Autodesk Fusion 360 part; units mm, degrees
note: some values were not read from the file. Set by a fixed rule: which sketch regions a step uses.
(part 2 of 2)
  spline S201 degree 3 poles (6.8488, 8.7661) (6.8423, 8.7918) (6.8421, 8.8259) (6.8482, 8.842) knots 0 0 0 0 1 1 1 1
  spline S202 degree 3 poles (8.7414, 7.2125) (8.7777, 7.2173) (8.7826, 7.2354) (8.7879, 7.3852) knots 0 0 0 0 1 1 1 1
  spline S203 degree 3 poles (9.5315, 7.0264) (9.6667, 6.9334) (9.8914, 6.6784) (9.9898, 6.5065) knots 0 0 0 0 1 1 1 1
  spline S204 degree 3 poles (9.748, 4.1018) (9.7258, 4.0149) (9.6698, 3.8347) (9.6236, 3.7012) knots 0 0 0 0 1 1 1 1
  spline S205 degree 3 poles (9.605, 10.5653) (9.605, 10.4649) (9.5312, 10.3126) (9.4656, 10.2775) knots 0 0 0 0 1 1 1 1
  spline S206 degree 3 poles (1.6447, 7.4321) (1.665, 7.8082) (1.7553, 8.1252) (1.9194, 8.3954) knots 0 0 0 0 1 1 1 1
  spline S207 degree 3 poles (9.5653, 3.7025) (9.6095, 3.8254) (9.6666, 4.0083) (9.6922, 4.1089) knots 0 0 0 0 1 1 1 1
  spline S208 degree 3 poles (9.4532, 3.3234) (9.4707, 3.409) (9.5212, 3.5795) (9.5653, 3.7025) knots 0 0 0 0 1 1 1 1
  spline S209 degree 3 poles (7.2255, 1.1728) (7.0951, 1.1191) (7.0078, 1.066) (6.9157, 0.9846) knots 0 0 0 0 1 1 1 1
  spline S210 degree 3 poles (10.2177, 5.0639) (10.1598, 4.8501) (10.0228, 4.569) (9.8929, 4.3977) knots 0 0 0 0 1 1 1 1
  spline S211 degree 3 poles (8.0403, 1.7091) (8.1353, 1.7773) (8.2598, 1.8521) (8.3169, 1.8754) knots 0 0 0 0 1 1 1 1
  spline S212 degree 3 poles (8.3787, 8.4165) (8.1204, 8.6765) (7.8311, 8.8118) (7.451, 8.8504) knots 0 0 0 0 1 1 1 1
  spline S213 degree 3 poles (8.0122, 1.6173) (7.7401, 1.4262) (7.4702, 1.2738) (7.2255, 1.1728) knots 0 0 0 0 1 1 1 1
  spline S214 degree 3 poles (1.4592, 7.0165) (1.6041, 7.1229) (1.6313, 7.1838) (1.6447, 7.4321) knots 0 0 0 0 1 1 1 1
  spline S215 degree 3 poles (6.8967, 8.8154) (6.8438, 8.7625) (7.1598, 8.3823) (7.5375, 8.0447) knots 0 0 0 0 1 1 1 1
  spline S216 degree 3 poles (9.404, 10.1458) (9.3772, 10.0264) (9.2567, 9.8669) (9.1498, 9.8097) knots 0 0 0 0 1 1 1 1
  spline S217 degree 3 poles (7.451, 8.8504) (7.2485, 8.871) (6.9323, 8.851) (6.8967, 8.8154) knots 0 0 0 0 1 1 1 1
  spline S218 degree 3 poles (2.0429, 7.257) (2.0099, 7.3294) (2.0562, 7.7293) (2.1195, 7.9187) knots 0 0 0 0 1 1 1 1
  spline S219 degree 3 poles (9.3549, 7.4617) (9.369, 7.1961) (9.4015, 7.1158) (9.5315, 7.0264) knots 0 0 0 0 1 1 1 1
  spline S220 degree 3 poles (8.7879, 7.3852) (8.7955, 7.6006) (8.7375, 7.8504) (8.6269, 8.0792) knots 0 0 0 0 1 1 1 1
  line L42 (8.5585, 7.2249) -> (8.5585, 7.2249)
  spline S221 degree 3 poles (9.7891, 11.6914) (9.7747, 11.6536) (9.7797, 11.6222) (9.8094, 11.5639) knots 0 0 0 0 1 1 1 1
  spline S222 degree 3 poles (9.1498, 9.8097) (9.1159, 9.7916) (9.0876, 9.7515) (9.0721, 9.6998) knots 0 0 0 0 1 1 1 1
  spline S223 degree 3 poles (2.481, 8.5) (2.6158, 8.635) (2.6801, 8.6816) (2.8384, 8.759) knots 0 0 0 0 1 1 1 1
  spline S224 degree 3 poles (10.2182, 5.9527) (10.2797, 5.7253) (10.2795, 5.292) (10.2177, 5.0639) knots 0 0 0 0 1 1 1 1
  line L43 (2.0249, 10.215) -> (2.1125, 10.2252)
  line L44 (5.7675, 7.7349) -> (5.7675, 7.7349)
  spline S225 degree 3 poles (1.477, 11.3964) (1.477, 11.406) (1.5272, 11.4139) (1.5887, 11.4139) knots 0 0 0 0 1 1 1 1
  spline S226 degree 3 poles (5.1964, 5.9716) (5.0404, 5.426) (4.5977, 4.9756) (4.075, 4.8308) knots 0 0 0 0 1 1 1 1
  spline S227 degree 3 poles (4.3387, 8.5706) (4.0922, 8.182) (4.6976, 7.738) (5.5003, 7.7186) knots 0 0 0 0 1 1 1 1
  spline S228 degree 3 poles (2.6301, 9.5918) (2.4593, 9.6417) (2.2491, 9.7435) (2.2491, 9.7763) knots 0 0 0 0 1 1 1 1
  spline S229 degree 3 poles (5.7675, 7.7349) (6.1571, 7.7759) (6.45, 7.8899) (6.6031, 8.0602) knots 0 0 0 0 1 1 1 1
  spline S230 degree 3 poles (2.003, 10.3004) (1.7807, 10.4532) (1.6559, 10.6247) (1.7891, 10.5945) knots 0 0 0 0 1 1 1 1
  spline S231 degree 3 poles (5.0939, 9.0802) (4.7717, 8.9797) (4.4682, 8.7749) (4.3387, 8.5706) knots 0 0 0 0 1 1 1 1
  spline S232 degree 3 poles (1.7972, 10.7093) (1.6781, 10.811) (1.5786, 10.9388) (1.5786, 10.9899) knots 0 0 0 0 1 1 1 1
  spline S233 degree 3 poles (5.0735, 5.7716) (5.1562, 5.9541) (5.1945, 6.1138) (5.208, 6.3339) knots 0 0 0 0 1 1 1 1
  spline S234 degree 3 poles (4.0117, 4.8607) (4.4627, 4.9671) (4.8653, 5.3124) (5.0735, 5.7716) knots 0 0 0 0 1 1 1 1
  spline S235 degree 3 poles (5.208, 6.3339) (5.2458, 6.9461) (4.8768, 7.4468) (4.3151, 7.5455) knots 0 0 0 0 1 1 1 1
  spline S236 degree 3 poles (4.3151, 7.5455) (4.1262, 7.5787) (3.9908, 7.5694) (3.7838, 7.5092) knots 0 0 0 0 1 1 1 1
  spline S237 degree 3 poles (8.2433, 6.7505) (8.3487, 6.5329) (8.3856, 6.3861) (8.3997, 6.1287) knots 0 0 0 0 1 1 1 1
  spline S238 degree 3 poles (7.5116, 7.5114) (7.8229, 7.3495) (8.0852, 7.0767) (8.2433, 6.7505) knots 0 0 0 0 1 1 1 1
  spline S239 degree 3 poles (2.2593, 9.929) (2.0696, 10.0329) (1.9188, 10.1485) (1.9297, 10.1816) knots 0 0 0 0 1 1 1 1
  spline S240 degree 3 poles (5.8117, 6.8927) (6.0456, 7.6034) (6.8041, 7.8795) (7.5116, 7.5114) knots 0 0 0 0 1 1 1 1
  spline S241 degree 3 poles (5.5003, 7.7186) (5.5506, 7.7174) (5.6708, 7.7247) (5.7675, 7.7349) knots 0 0 0 0 1 1 1 1
  spline S242 degree 3 poles (3.7122, 4.831) (3.8072, 4.8309) (3.942, 4.8443) (4.0117, 4.8607) knots 0 0 0 0 1 1 1 1
  spline S243 degree 3 poles (1.7003, 11.4393) (1.7, 11.4746) (1.6076, 11.6698) (1.5583, 11.7389) knots 0 0 0 0 1 1 1 1
  spline S244 degree 3 poles (8.3997, 6.1287) (8.4213, 5.7357) (8.311, 5.4218) (8.0651, 5.1759) knots 0 0 0 0 1 1 1 1
  spline S245 degree 3 poles (4.279, 8.5648) (4.3224, 8.6498) (4.4952, 8.8262) (4.6141, 8.9068) knots 0 0 0 0 1 1 1 1
  spline S246 degree 3 poles (8.0651, 5.1759) (7.7847, 4.8955) (7.4026, 4.7916) (6.9851, 4.8821) knots 0 0 0 0 1 1 1 1
  spline S247 degree 3 poles (7.8704, 7.193) (7.1638, 7.8887) (6.1547, 7.7346) (5.8598, 6.8859) knots 0 0 0 0 1 1 1 1
  spline S248 degree 3 poles (8.3349, 5.7751) (8.4358, 6.2558) (8.2518, 6.8174) (7.8704, 7.193) knots 0 0 0 0 1 1 1 1
  spline S249 degree 3 poles (6.6831, 8.5182) (6.5678, 8.7465) (6.2355, 8.9773) (5.872, 9.0815) knots 0 0 0 0 1 1 1 1
  spline S250 degree 3 poles (2.0867, 7.5233) (2.0579, 7.2435) (2.0842, 7.2071) (2.2619, 7.281) knots 0 0 0 0 1 1 1 1
  spline S251 degree 3 poles (6.7094, 8.5665) (6.7799, 8.4383) (6.7915, 8.2563) (6.7359, 8.1525) knots 0 0 0 0 1 1 1 1
  spline S252 degree 3 poles (2.7063, 9.5038) (2.7343, 9.5144) (2.7571, 9.5302) (2.7571, 9.5389) knots 0 0 0 0 1 1 1 1
  spline S253 degree 3 poles (6.7359, 8.1525) (6.5514, 7.8081) (5.9013, 7.6142) (5.2158, 7.6991) knots 0 0 0 0 1 1 1 1
  spline S254 degree 3 poles (2.7571, 9.5389) (2.7571, 9.5475) (2.6999, 9.5713) (2.6301, 9.5918) knots 0 0 0 0 1 1 1 1
  spline S255 degree 3 poles (1.9297, 10.1816) (1.9339, 10.1944) (1.9767, 10.2094) (2.0249, 10.215) knots 0 0 0 0 1 1 1 1
  spline S256 degree 3 poles (5.1947, 9.1494) (5.4148, 9.1938) (5.7145, 9.1806) (5.9169, 9.1174) knots 0 0 0 0 1 1 1 1
  spline S257 degree 3 poles (2.2491, 9.7763) (2.2491, 9.7911) (2.2874, 9.8111) (2.3355, 9.8214) knots 0 0 0 0 1 1 1 1
  spline S258 degree 3 poles (5.9169, 9.1174) (6.2615, 9.0098) (6.592, 8.7801) (6.7094, 8.5665) knots 0 0 0 0 1 1 1 1
  spline S259 degree 3 poles (1.5887, 11.4139) (1.6647, 11.4139) (1.7004, 11.422) (1.7003, 11.4393) knots 0 0 0 0 1 1 1 1
  spline S260 degree 3 poles (3.7934, 7.5652) (3.9997, 7.6214) (4.3135, 7.6144) (4.4966, 7.5495) knots 0 0 0 0 1 1 1 1
  spline S261 degree 3 poles (5.2283, 6.6997) (5.2698, 6.5029) (5.2557, 6.1786) (5.1964, 5.9716) knots 0 0 0 0 1 1 1 1
  spline S262 degree 3 poles (1.698, 11.1132) (1.5887, 11.2162) (1.477, 11.3594) (1.477, 11.3964) knots 0 0 0 0 1 1 1 1
  spline S263 degree 3 poles (4.4966, 7.5495) (4.8766, 7.4147) (5.1424, 7.106) (5.2283, 6.6997) knots 0 0 0 0 1 1 1 1
  spline S264 degree 3 poles (4.075, 4.8308) (3.9008, 4.7825) (3.5773, 4.7772) (3.4214, 4.8201) knots 0 0 0 0 1 1 1 1
  spline S265 degree 3 poles (3.9654, 8.7696) (4.0196, 8.8762) (3.9969, 8.8841) (3.635, 8.8841) knots 0 0 0 0 1 1 1 1
  spline S266 degree 3 poles (6.6031, 8.0602) (6.7405, 8.213) (6.7654, 8.3552) (6.6831, 8.5182) knots 0 0 0 0 1 1 1 1
  spline S267 degree 3 poles (3.7838, 7.5092) (3.1288, 7.3184) (2.6508, 6.6827) (2.6479, 5.9986) knots 0 0 0 0 1 1 1 1
  spline S268 degree 3 poles (2.7689, 5.4275) (2.9421, 5.0611) (3.3051, 4.8316) (3.7122, 4.831) knots 0 0 0 0 1 1 1 1
  spline S269 degree 3 poles (1.5786, 10.9899) (1.5786, 11.0151) (1.6007, 11.0195) (1.6954, 11.0133) knots 0 0 0 0 1 1 1 1
  spline S270 degree 3 poles (2.6479, 5.9986) (2.6469, 5.76) (2.6754, 5.6251) (2.7689, 5.4275) knots 0 0 0 0 1 1 1 1
  spline S271 degree 3 poles (5.802, 6.0703) (5.7337, 6.3243) (5.7377, 6.668) (5.8117, 6.8927) knots 0 0 0 0 1 1 1 1
  spline S272 degree 3 poles (6.9851, 4.8821) (6.4518, 4.9978) (5.9569, 5.4948) (5.802, 6.0703) knots 0 0 0 0 1 1 1 1
  spline S273 degree 3 poles (3.1867, 9.2589) (3.2684, 9.3193) (3.2462, 9.3318) (3.0249, 9.3504) knots 0 0 0 0 1 1 1 1
  spline S274 degree 3 poles (4.5847, 7.9094) (4.4511, 7.9906) (4.3109, 8.1351) (4.2694, 8.2344) knots 0 0 0 0 1 1 1 1
  spline S275 degree 3 poles (3.635, 8.8841) (3.3624, 8.8841) (3.2924, 8.8773) (3.1545, 8.8373) knots 0 0 0 0 1 1 1 1
  spline S276 degree 3 poles (3.0249, 9.3504) (2.7221, 9.3759) (2.5667, 9.4507) (2.7063, 9.5038) knots 0 0 0 0 1 1 1 1
  spline S277 degree 3 poles (4.6141, 8.9068) (4.7582, 9.0046) (5.0205, 9.1142) (5.1947, 9.1494) knots 0 0 0 0 1 1 1 1
  spline S278 degree 3 poles (4.2694, 8.2344) (4.2291, 8.3308) (4.2333, 8.4754) (4.279, 8.5648) knots 0 0 0 0 1 1 1 1
  spline S279 degree 3 poles (5.2158, 7.6991) (5.0217, 7.7232) (4.7329, 7.8194) (4.5847, 7.9094) knots 0 0 0 0 1 1 1 1
  spline S280 degree 3 poles (3.1584, 9.1724) (3.1077, 9.1856) (3.1141, 9.2052) (3.1867, 9.2589) knots 0 0 0 0 1 1 1 1
  spline S281 degree 3 poles (1.7891, 10.5945) (1.813, 10.5891) (1.8498, 10.5912) (1.8708, 10.5992) knots 0 0 0 0 1 1 1 1
  line L45 (2.3355, 9.8214) -> (2.4218, 9.84)
  line L46 (2.4218, 9.84) -> (2.2593, 9.929)
  spline S282 degree 3 poles (5.872, 9.0815) (5.6441, 9.1468) (5.3056, 9.1463) (5.0939, 9.0802) knots 0 0 0 0 1 1 1 1
  spline S283 degree 3 poles (1.8708, 10.5992) (1.9038, 10.6117) (1.8936, 10.6269) (1.7972, 10.7093) knots 0 0 0 0 1 1 1 1
  line L47 (2.1125, 10.2252) -> (2.003, 10.3004)
  spline S284 degree 3 poles (1.2763, 4.8425) (1.0557, 5.2885) (1.0727, 5.8763) (1.318, 6.288) knots 0 0 0 0 1 1 1 1
  spline S285 degree 3 poles (4.2059, 3.3632) (4.1426, 3.5277) (4.1196, 3.8574) (4.1584, 4.0441) knots 0 0 0 0 1 1 1 1
  spline S286 degree 3 poles (4.1795, 1.601) (4.1795, 1.5168) (4.292, 1.3626) (4.4437, 1.2387) knots 0 0 0 0 1 1 1 1
  spline S287 degree 3 poles (8.7941, 4.5029) (8.5375, 4.6444) (8.1575, 4.4807) (7.7149, 4.0381) knots 0 0 0 0 1 1 1 1
  spline S288 degree 3 poles (1.8517, 3.8425) (1.9024, 4.3071) (2.1479, 4.4859) (2.5803, 4.3732) knots 0 0 0 0 1 1 1 1
  spline S289 degree 3 poles (5.1369, 0.8861) (5.3563, 0.8305) (5.6964, 0.8433) (5.9169, 0.9154) knots 0 0 0 0 1 1 1 1
  spline S290 degree 3 poles (3.8769, 2.6151) (3.876, 3.0027) (3.6864, 3.4542) (3.3879, 3.7794) knots 0 0 0 0 1 1 1 1
  spline S291 degree 3 poles (7.7149, 4.0381) (7.3234, 3.6464) (7.1023, 3.2168) (7.0405, 2.7271) knots 0 0 0 0 1 1 1 1
  spline S292 degree 3 poles (5.8166, 2.5154) (5.6571, 2.4863) (5.3575, 2.4901) (5.2057, 2.5232) knots 0 0 0 0 1 1 1 1
  spline S293 degree 3 poles (7.573, 2.0081) (7.5003, 2.0091) (7.4064, 2.0179) (7.3644, 2.0278) knots 0 0 0 0 1 1 1 1
  spline S294 degree 3 poles (5.3561, 5.0161) (5.0183, 4.9711) (4.7676, 4.8493) (4.535, 4.6169) knots 0 0 0 0 1 1 1 1
  spline S295 degree 3 poles (1.9337, 6.8216) (2.033, 6.8216) (2.1149, 6.7355) (2.1628, 6.5806) knots 0 0 0 0 1 1 1 1
  spline S296 degree 3 poles (7.3644, 2.0278) (7.1255, 2.0841) (7.0192, 2.2134) (6.9918, 2.481) knots 0 0 0 0 1 1 1 1
  spline S297 degree 3 poles (6.0735, 4.9732) (6.4565, 4.8291) (6.793, 4.4636) (6.8905, 4.0856) knots 0 0 0 0 1 1 1 1
  spline S298 degree 3 poles (6.8925, 3.4832) (6.7694, 3.0106) (6.3214, 2.6076) (5.8166, 2.5154) knots 0 0 0 0 1 1 1 1
  spline S299 degree 3 poles (1.318, 6.288) (1.4705, 6.544) (1.7908, 6.8216) (1.9337, 6.8216) knots 0 0 0 0 1 1 1 1
  spline S300 degree 3 poles (2.0553, 3.0208) (2.3171, 2.4001) (3.0728, 1.9597) (3.605, 2.1177) knots 0 0 0 0 1 1 1 1
  spline S301 degree 3 poles (7.0405, 2.7271) (7.0203, 2.5675) (7.0217, 2.5209) (7.0501, 2.406) knots 0 0 0 0 1 1 1 1
  spline S302 degree 3 poles (2.1628, 6.5806) (2.2177, 6.4035) (2.2111, 5.7963) (2.1508, 5.4703) knots 0 0 0 0 1 1 1 1
  spline S303 degree 3 poles (1.7774, 4.4944) (1.7039, 4.4325) (1.6036, 4.4287) (1.532, 4.485) knots 0 0 0 0 1 1 1 1
  spline S304 degree 3 poles (2.1508, 5.4703) (2.0653, 5.0077) (1.9123, 4.6079) (1.7774, 4.4944) knots 0 0 0 0 1 1 1 1
  spline S305 degree 3 poles (2.0662, 6.6896) (1.9763, 6.835) (1.8403, 6.7946) (1.5886, 6.5476) knots 0 0 0 0 1 1 1 1
  spline S306 degree 3 poles (1.5886, 6.5476) (1.3126, 6.2766) (1.1918, 5.9956) (1.1766, 5.5888) knots 0 0 0 0 1 1 1 1
  spline S307 degree 3 poles (1.7632, 4.5506) (2.089, 4.8764) (2.2937, 6.3214) (2.0662, 6.6896) knots 0 0 0 0 1 1 1 1
  spline S308 degree 3 poles (1.315, 4.8721) (1.4069, 4.682) (1.5781, 4.4848) (1.6511, 4.4848) knots 0 0 0 0 1 1 1 1
  spline S309 degree 3 poles (7.5304, 4.9225) (7.9305, 5.0168) (8.2458, 5.351) (8.3349, 5.7751) knots 0 0 0 0 1 1 1 1
  spline S310 degree 3 poles (8.9565, 4.4076) (9.1428, 4.1139) (9.1825, 3.5377) (9.0446, 3.127) knots 0 0 0 0 1 1 1 1
  spline S311 degree 3 poles (8.5658, 2.5023) (8.9324, 2.8542) (9.0801, 3.1912) (9.0784, 3.6716) knots 0 0 0 0 1 1 1 1
  spline S312 degree 3 poles (8.2411, 4.5037) (8.5457, 4.6572) (8.8217, 4.6201) (8.9565, 4.4076) knots 0 0 0 0 1 1 1 1
  spline S313 degree 3 poles (5.2057, 2.5232) (4.7454, 2.6236) (4.3684, 2.9404) (4.2059, 3.3632) knots 0 0 0 0 1 1 1 1
  spline S314 degree 3 poles (5.2033, 2.0675) (4.6459, 1.9977) (4.1795, 1.7851) (4.1795, 1.601) knots 0 0 0 0 1 1 1 1
  spline S315 degree 3 poles (9.0446, 3.127) (8.9827, 2.9425) (8.9388, 2.8664) (8.7732, 2.6561) knots 0 0 0 0 1 1 1 1
  spline S316 degree 3 poles (6.0712, 5.5887) (6.4202, 5.0771) (7.0217, 4.8025) (7.5304, 4.9225) knots 0 0 0 0 1 1 1 1
  spline S317 degree 3 poles (5.8598, 6.8859) (5.7226, 6.4907) (5.8063, 5.9769) (6.0712, 5.5887) knots 0 0 0 0 1 1 1 1
  spline S318 degree 3 poles (3.9151, 2.4514) (3.8644, 2.1505) (3.7196, 2.0451) (3.3609, 2.0478) knots 0 0 0 0 1 1 1 1
  spline S319 degree 3 poles (2.5803, 4.3732) (2.9431, 4.2787) (3.4539, 3.8602) (3.6698, 3.4806) knots 0 0 0 0 1 1 1 1
  spline S320 degree 3 poles (3.6698, 3.4806) (3.8572, 3.151) (3.9602, 2.7188) (3.9151, 2.4514) knots 0 0 0 0 1 1 1 1
  spline S321 degree 3 poles (9.0784, 3.6716) (9.0769, 4.0782) (8.9637, 4.4094) (8.7941, 4.5029) knots 0 0 0 0 1 1 1 1
  spline S322 degree 3 poles (7.0501, 2.406) (7.0914, 2.2385) (7.1311, 2.1768) (7.2303, 2.1262) knots 0 0 0 0 1 1 1 1
  spline S323 degree 3 poles (8.5585, 7.2249) (8.0487, 7.4667) (6.9194, 8.4847) (6.8488, 8.7661) knots 0 0 0 0 1 1 1 1
  spline S324 degree 3 poles (3.3609, 2.0478) (3.2458, 2.0487) (3.1245, 2.0633) (3.046, 2.0858) knots 0 0 0 0 1 1 1 1
  spline S325 degree 3 poles (3.3879, 3.7794) (3.133, 4.0572) (2.7638, 4.2919) (2.4977, 4.3455) knots 0 0 0 0 1 1 1 1
  spline S326 degree 3 poles (6.9918, 2.481) (6.9569, 2.8215) (7.1182, 3.3418) (7.3767, 3.7227) knots 0 0 0 0 1 1 1 1
  spline S327 degree 3 poles (3.605, 2.1177) (3.798, 2.175) (3.8775, 2.3205) (3.8769, 2.6151) knots 0 0 0 0 1 1 1 1
  spline S328 degree 3 poles (2.4977, 4.3455) (2.3974, 4.3657) (2.3457, 4.366) (2.2539, 4.3467) knots 0 0 0 0 1 1 1 1
  spline S329 degree 3 poles (1.9805, 4.1384) (1.8435, 3.8636) (1.8706, 3.4587) (2.0553, 3.0208) knots 0 0 0 0 1 1 1 1
  spline S330 degree 3 poles (4.1584, 4.0441) (4.2476, 4.4737) (4.6319, 4.8671) (5.1041, 5.0121) knots 0 0 0 0 1 1 1 1
  spline S331 degree 3 poles (6.8905, 4.0856) (6.931, 3.9285) (6.932, 3.6349) (6.8925, 3.4832) knots 0 0 0 0 1 1 1 1
  line L48 (3.605, 2.1177) -> (3.605, 2.1177)
  spline S332 degree 3 poles (5.1041, 5.0121) (5.3932, 5.1009) (5.7746, 5.0856) (6.0735, 4.9732) knots 0 0 0 0 1 1 1 1
  spline S333 degree 3 poles (5.8636, 2.5751) (6.3479, 2.6912) (6.7466, 3.0695) (6.8508, 3.5115) knots 0 0 0 0 1 1 1 1
  spline S334 degree 3 poles (6.8508, 3.5115) (6.9928, 4.1138) (6.633, 4.7275) (6.011, 4.9438) knots 0 0 0 0 1 1 1 1
  spline S335 degree 3 poles (6.011, 4.9438) (5.7894, 5.0209) (5.572, 5.0449) (5.3561, 5.0161) knots 0 0 0 0 1 1 1 1
  spline S336 degree 3 poles (4.535, 4.6169) (3.9096, 3.992) (4.137, 2.9982) (4.9874, 2.6389) knots 0 0 0 0 1 1 1 1
  spline S337 degree 3 poles (1.532, 4.485) (1.46, 4.5417) (1.3469, 4.6998) (1.2763, 4.8425) knots 0 0 0 0 1 1 1 1
  spline S338 degree 3 poles (4.9874, 2.6389) (5.2441, 2.5305) (5.5763, 2.5063) (5.8636, 2.5751) knots 0 0 0 0 1 1 1 1
  spline S339 degree 3 poles (7.8229, 2.0793) (8.106, 2.1431) (8.3164, 2.2629) (8.5658, 2.5023) knots 0 0 0 0 1 1 1 1
  spline S340 degree 3 poles (3.046, 2.0858) (2.6648, 2.1948) (2.2372, 2.5427) (2.0636, 2.8851) knots 0 0 0 0 1 1 1 1
  spline S341 degree 3 poles (7.2303, 2.1262) (7.3945, 2.0425) (7.5904, 2.0269) (7.8229, 2.0793) knots 0 0 0 0 1 1 1 1
  spline S342 degree 3 poles (7.3767, 3.7227) (7.5602, 3.9932) (7.9793, 4.3719) (8.2411, 4.5037) knots 0 0 0 0 1 1 1 1
  spline S343 degree 3 poles (2.0636, 2.8851) (1.9169, 3.1746) (1.8244, 3.5925) (1.8517, 3.8425) knots 0 0 0 0 1 1 1 1
  spline S344 degree 3 poles (4.4437, 1.2387) (4.6081, 1.1045) (4.9387, 0.9364) (5.1369, 0.8861) knots 0 0 0 0 1 1 1 1
  spline S345 degree 3 poles (2.2539, 4.3467) (2.1024, 4.315) (2.0478, 4.2735) (1.9805, 4.1384) knots 0 0 0 0 1 1 1 1
  spline S346 degree 3 poles (8.7732, 2.6561) (8.4493, 2.2449) (8.0006, 2.0027) (7.573, 2.0081) knots 0 0 0 0 1 1 1 1
  spline S347 degree 3 poles (2.2627, 12.3324) (2.2362, 12.3084) (2.1829, 12.2975) (2.0784, 12.2949) knots 0 0 0 0 1 1 1 1
  spline S348 degree 3 poles (2.2515, 8.7013) (1.9092, 8.3763) (1.745, 8.0027) (1.7001, 7.4465) knots 0 0 0 0 1 1 1 1
  spline S349 degree 3 poles (1.536, 6.9964) (1.3577, 6.8911) (1.1284, 6.6154) (0.9933, 6.3441) knots 0 0 0 0 1 1 1 1
  spline S350 degree 3 poles (1.1586, 4.4335) (1.2366, 4.3313) (1.2747, 4.2591) (1.2927, 4.1795) knots 0 0 0 0 1 1 1 1
  spline S351 degree 3 poles (4.1687, 12.3626) (4.1188, 12.3545) (4.0743, 12.3646) (4.0106, 12.3984) knots 0 0 0 0 1 1 1 1
  spline S352 degree 3 poles (1.2628, 11.2412) (1.3046, 11.1731) (1.3107, 11.1432) (1.301, 11.0568) knots 0 0 0 0 1 1 1 1
  spline S353 degree 3 poles (0.9933, 6.3441) (0.6714, 5.6974) (0.7324, 4.9921) (1.1586, 4.4335) knots 0 0 0 0 1 1 1 1
  spline S354 degree 3 poles (9.3892, 4.6308) (9.6325, 4.9089) (9.7597, 5.3563) (9.7064, 5.7459) knots 0 0 0 0 1 1 1 1
  spline S355 degree 3 poles (1.2552, 11.5544) (1.1977, 11.4601) (1.2006, 11.3427) (1.2628, 11.2412) knots 0 0 0 0 1 1 1 1
  spline S356 degree 3 poles (6.7938, 1.7083) (6.7448, 1.8302) (6.5104, 1.9507) (6.1709, 2.0287) knots 0 0 0 0 1 1 1 1
  spline S357 degree 3 poles (2.5095, 12.4097) (2.4034, 12.4096) (2.3187, 12.383) (2.2627, 12.3324) knots 0 0 0 0 1 1 1 1
  spline S358 degree 3 poles (6.1709, 2.0287) (5.9404, 2.0816) (5.4672, 2.1006) (5.2033, 2.0675) knots 0 0 0 0 1 1 1 1
  spline S359 degree 3 poles (2.0784, 12.2949) (1.9104, 12.2908) (1.8123, 12.2563) (1.7214, 12.1694) knots 0 0 0 0 1 1 1 1
  spline S360 degree 3 poles (1.301, 11.0568) (1.2885, 10.9465) (1.3132, 10.8774) (1.4111, 10.7486) knots 0 0 0 0 1 1 1 1
  spline S361 degree 3 poles (6.4208, 1.1158) (6.1042, 0.9011) (5.8117, 0.8062) (5.4726, 0.8082) knots 0 0 0 0 1 1 1 1
  spline S362 degree 3 poles (1.5759, 3.2199) (1.6565, 2.8674) (1.9003, 2.4622) (2.1812, 2.2139) knots 0 0 0 0 1 1 1 1
  spline S363 degree 3 poles (1.4266, 3.7329) (1.4864, 3.5485) (1.5536, 3.3177) (1.5759, 3.2199) knots 0 0 0 0 1 1 1 1
  spline S364 degree 3 poles (1.2927, 4.1795) (1.3066, 4.1183) (1.3669, 3.9173) (1.4266, 3.7329) knots 0 0 0 0 1 1 1 1
  spline S365 degree 3 poles (2.6248, 5.7149) (2.5753, 5.9926) (2.5926, 6.2105) (2.6869, 6.4974) knots 0 0 0 0 1 1 1 1
  spline S366 degree 3 poles (6.7679, 1.5412) (6.8139, 1.6334) (6.8166, 1.6513) (6.7938, 1.7083) knots 0 0 0 0 1 1 1 1
  spline S367 degree 3 poles (2.1812, 2.2139) (2.3482, 2.0664) (2.5742, 1.9151) (2.6946, 1.8701) knots 0 0 0 0 1 1 1 1
  spline S368 degree 3 poles (2.6946, 1.8701) (2.7457, 1.851) (2.879, 1.7704) (2.9908, 1.6908) knots 0 0 0 0 1 1 1 1
  spline S369 degree 3 poles (8.9493, 6.8622) (9.0141, 6.8622) (9.1957, 6.7465) (9.3275, 6.6214) knots 0 0 0 0 1 1 1 1
  spline S370 degree 3 poles (9.7064, 5.7459) (9.6484, 6.1694) (9.4304, 6.525) (9.0903, 6.7508) knots 0 0 0 0 1 1 1 1
  spline S371 degree 3 poles (8.7231, 6.1205) (8.7265, 5.6296) (8.8314, 5.1128) (8.9961, 4.7755) knots 0 0 0 0 1 1 1 1
  spline S372 degree 3 poles (8.9961, 4.7755) (9.1342, 4.4929) (9.2359, 4.4555) (9.3892, 4.6308) knots 0 0 0 0 1 1 1 1
  spline S373 degree 3 poles (2.6869, 6.4974) (2.7845, 6.794) (3.0301, 7.132) (3.2831, 7.3177) knots 0 0 0 0 1 1 1 1
  spline S374 degree 3 poles (8.9188, 6.8096) (8.7786, 6.7603) (8.7202, 6.5546) (8.7231, 6.1205) knots 0 0 0 0 1 1 1 1
  spline S375 degree 3 poles (4.4915, 12.2462) (4.3747, 12.353) (4.2923, 12.3827) (4.1687, 12.3626) knots 0 0 0 0 1 1 1 1
  spline S376 degree 3 poles (3.0681, 12.4687) (3.0415, 12.4808) (2.9721, 12.496) (2.9138, 12.5025) knots 0 0 0 0 1 1 1 1
  spline S377 degree 3 poles (1.8606, 9.8776) (1.9316, 9.8246) (1.9664, 9.7814) (1.9832, 9.7251) knots 0 0 0 0 1 1 1 1
  spline S378 degree 3 poles (3.4214, 4.8201) (3.0206, 4.9303) (2.7005, 5.2898) (2.6248, 5.7149) knots 0 0 0 0 1 1 1 1
  spline S379 degree 3 poles (1.2643, 11.7295) (1.2964, 11.6274) (1.2961, 11.6214) (1.2552, 11.5544) knots 0 0 0 0 1 1 1 1
  spline S380 degree 3 poles (5.9169, 0.9154) (6.2637, 1.0289) (6.6566, 1.3178) (6.7679, 1.5412) knots 0 0 0 0 1 1 1 1
  spline S381 degree 3 poles (9.0903, 6.7508) (8.9905, 6.817) (8.9649, 6.8258) (8.9188, 6.8096) knots 0 0 0 0 1 1 1 1
  spline S382 degree 3 poles (9.1455, 4.5032) (8.9801, 4.604) (8.825, 4.9817) (8.7276, 5.5211) knots 0 0 0 0 1 1 1 1
  spline S383 degree 3 poles (1.6511, 4.4848) (1.6765, 4.4848) (1.727, 4.5144) (1.7632, 4.5506) knots 0 0 0 0 1 1 1 1
  spline S384 degree 3 poles (6.8522, 1.698) (6.8819, 1.563) (6.6817, 1.2929) (6.4208, 1.1158) knots 0 0 0 0 1 1 1 1
  spline S385 degree 3 poles (3.721, 12.4524) (3.6576, 12.4349) (3.6268, 12.4395) (3.5231, 12.4816) knots 0 0 0 0 1 1 1 1
  spline S386 degree 3 poles (9.6023, 4.8733) (9.5129, 4.6884) (9.3189, 4.4644) (9.2484, 4.4645) knots 0 0 0 0 1 1 1 1
  spline S387 degree 3 poles (1.5577, 12.1079) (1.3135, 12.106) (1.1942, 11.9522) (1.2643, 11.7295) knots 0 0 0 0 1 1 1 1
  spline S388 degree 3 poles (5.4726, 0.8082) (5.3444, 0.809) (5.1979, 0.8223) (5.1346, 0.839) knots 0 0 0 0 1 1 1 1
  spline S389 degree 3 poles (8.7176, 6.6068) (8.763, 6.754) (8.8612, 6.8622) (8.9493, 6.8622) knots 0 0 0 0 1 1 1 1
  spline S390 degree 3 poles (1.6459, 10.1868) (1.6625, 10.08) (1.7411, 9.9668) (1.8606, 9.8776) knots 0 0 0 0 1 1 1 1
  spline S391 degree 3 poles (2.7234, 9.0482) (2.6399, 9.0161) (2.3883, 8.8312) (2.2515, 8.7013) knots 0 0 0 0 1 1 1 1
  spline S392 degree 3 poles (1.1766, 5.5888) (1.1653, 5.2872) (1.1993, 5.1114) (1.315, 4.8721) knots 0 0 0 0 1 1 1 1
  spline S393 degree 3 poles (2.9138, 12.5025) (2.8254, 12.5124) (2.7912, 12.5057) (2.7063, 12.4621) knots 0 0 0 0 1 1 1 1
  spline S394 degree 3 poles (1.4111, 10.7486) (1.4452, 10.7038) (1.4574, 10.6677) (1.4493, 10.6356) knots 0 0 0 0 1 1 1 1
  spline S395 degree 3 poles (1.4493, 10.6356) (1.43, 10.5588) (1.4747, 10.4401) (1.5568, 10.3501) knots 0 0 0 0 1 1 1 1
  spline S396 degree 3 poles (3.1955, 12.4891) (3.1318, 12.4549) (3.107, 12.4509) (3.0681, 12.4687) knots 0 0 0 0 1 1 1 1
  spline S397 degree 3 poles (1.7001, 7.4465) (1.6768, 7.1588) (1.6401, 7.0579) (1.536, 6.9964) knots 0 0 0 0 1 1 1 1
  spline S398 degree 3 poles (4.0106, 12.3984) (3.8907, 12.4622) (3.8105, 12.4771) (3.721, 12.4524) knots 0 0 0 0 1 1 1 1
  spline S399 degree 3 poles (2.7063, 12.4621) (2.6399, 12.4278) (2.5718, 12.4097) (2.5095, 12.4097) knots 0 0 0 0 1 1 1 1
  spline S400 degree 3 poles (1.5568, 10.3501) (1.6069, 10.295) (1.6378, 10.2384) (1.6459, 10.1868) knots 0 0 0 0 1 1 1 1
  spline S401 degree 3 poles (9.3275, 6.6214) (9.7762, 6.1953) (9.8903, 5.4691) (9.6023, 4.8733) knots 0 0 0 0 1 1 1 1
  spline S402 degree 3 poles (8.7276, 5.5211) (8.6688, 5.8465) (8.6634, 6.4313) (8.7176, 6.6068) knots 0 0 0 0 1 1 1 1
  spline S403 degree 3 poles (2.2501, 9.473) (2.3335, 9.4453) (2.3548, 9.4269) (2.3916, 9.351) knots 0 0 0 0 1 1 1 1
  spline S404 degree 3 poles (1.9832, 9.7251) (2.0143, 9.6213) (2.1285, 9.5134) (2.2501, 9.473) knots 0 0 0 0 1 1 1 1
  spline S405 degree 3 poles (3.2831, 7.3177) (3.4154, 7.4148) (3.6383, 7.5229) (3.7934, 7.5652) knots 0 0 0 0 1 1 1 1
  spline S406 degree 3 poles (9.2484, 4.4645) (9.2266, 4.4646) (9.1803, 4.482) (9.1455, 4.5032) knots 0 0 0 0 1 1 1 1
  spline S407 degree 3 poles (3.5231, 12.4816) (3.373, 12.5426) (3.2986, 12.5443) (3.1955, 12.4891) knots 0 0 0 0 1 1 1 1
  spline S408 degree 3 poles (1.7214, 12.1694) (1.6688, 12.1191) (1.6406, 12.1085) (1.5577, 12.1079) knots 0 0 0 0 1 1 1 1
  spline S409 degree 3 poles (2.3916, 9.351) (2.4401, 9.2507) (2.5193, 9.1932) (2.6612, 9.1553) knots 0 0 0 0 1 1 1 1
  spline S410 degree 3 poles (2.6612, 9.1553) (2.7606, 9.1287) (2.7921, 9.0745) (2.7234, 9.0482) knots 0 0 0 0 1 1 1 1
  spline S411 degree 3 poles (9.7496, 11.5514) (9.7096, 11.6298) (9.709, 11.6392) (9.7388, 11.7223) knots 0 0 0 0 1 1 1 1
  spline S412 degree 3 poles (9.554, 10.6423) (9.546, 10.6675) (9.5594, 10.7057) (9.5911, 10.7481) knots 0 0 0 0 1 1 1 1
  spline S413 degree 3 poles (7.264, 12.4551) (7.1823, 12.4738) (7.1593, 12.4702) (7.0552, 12.4225) knots 0 0 0 0 1 1 1 1
  spline S414 degree 3 poles (7.0552, 12.4225) (6.9703, 12.3837) (6.9048, 12.3689) (6.8167, 12.3689) knots 0 0 0 0 1 1 1 1
  spline S415 degree 3 poles (9.5911, 10.7481) (9.6874, 10.8767) (9.7122, 10.9468) (9.6995, 11.0543) knots 0 0 0 0 1 1 1 1
  spline S416 degree 3 poles (3.9052, 1.182) (3.9681, 1.1588) (4.0567, 1.0985) (4.1379, 1.0234) knots 0 0 0 0 1 1 1 1
  spline S417 degree 3 poles (5.4131, 11.2903) (5.309, 11.5849) (5.0924, 11.9007) (4.8843, 12.0613) knots 0 0 0 0 1 1 1 1
  spline S418 degree 3 poles (4.1389, 1.5972) (4.1389, 1.714) (4.2257, 1.8047) (4.4338, 1.9054) knots 0 0 0 0 1 1 1 1
  spline S419 degree 3 poles (8.6121, 9.3531) (8.6453, 9.4282) (8.6642, 9.4443) (8.7532, 9.4739) knots 0 0 0 0 1 1 1 1
  spline S420 degree 3 poles (9.0615, 8.3174) (8.9592, 8.5051) (8.6545, 8.813) (8.4213, 8.9643) knots 0 0 0 0 1 1 1 1
  spline S421 degree 3 poles (8.5039, 12.4097) (8.4291, 12.4097) (8.3652, 12.4253) (8.296, 12.4605) knots 0 0 0 0 1 1 1 1
  spline S422 degree 3 poles (7.4851, 12.4828) (7.3733, 12.4407) (7.3433, 12.4369) (7.264, 12.4551) knots 0 0 0 0 1 1 1 1
  spline S423 degree 3 poles (6.8167, 12.3689) (6.6714, 12.3689) (6.5908, 12.3342) (6.4852, 12.226) knots 0 0 0 0 1 1 1 1
  spline S424 degree 3 poles (6.3212, 12.1454) (6.2515, 12.1454) (6.2133, 12.1285) (6.1124, 12.0526) knots 0 0 0 0 1 1 1 1
  spline S425 degree 3 poles (5.5602, 11.2158) (5.5203, 11.0816) (5.4795, 11.1023) (5.4131, 11.2903) knots 0 0 0 0 1 1 1 1
  spline S426 degree 3 poles (4.6885, 12.1454) (4.6129, 12.1454) (4.5876, 12.1583) (4.4915, 12.2462) knots 0 0 0 0 1 1 1 1
  spline S427 degree 3 poles (5.0838, 0.5141) (5.2967, 0.4672) (5.8248, 0.4822) (6.0251, 0.5408) knots 0 0 0 0 1 1 1 1
  spline S428 degree 3 poles (8.7532, 9.4739) (8.8757, 9.5146) (8.9806, 9.613) (9.0186, 9.7228) knots 0 0 0 0 1 1 1 1
  spline S429 degree 3 poles (6.1794, 10.1542) (6.1427, 10.1539) (5.9718, 10.2754) (5.9163, 10.3413) knots 0 0 0 0 1 1 1 1
  spline S430 degree 3 poles (6.4382, 10.332) (6.3079, 10.2344) (6.1915, 10.1544) (6.1794, 10.1542) knots 0 0 0 0 1 1 1 1
  spline S431 degree 3 poles (5.9163, 10.3413) (5.7979, 10.4821) (5.7746, 10.5547) (5.7746, 10.784) knots 0 0 0 0 1 1 1 1
  spline S432 degree 3 poles (5.7746, 10.784) (5.7746, 10.9683) (5.7825, 11.0188) (5.8327, 11.1553) knots 0 0 0 0 1 1 1 1
  spline S433 degree 3 poles (8.9223, 12.2949) (8.8207, 12.2975) (8.7637, 12.3087) (8.738, 12.3312) knots 0 0 0 0 1 1 1 1
  spline S434 degree 3 poles (7.9821, 12.4796) (7.8808, 12.4495) (7.8727, 12.45) (7.8084, 12.4898) knots 0 0 0 0 1 1 1 1
  spline S435 degree 3 poles (6.3538, 11.8623) (6.3538, 11.8518) (6.3632, 11.8183) (6.3748, 11.7879) knots 0 0 0 0 1 1 1 1
  spline S436 degree 3 poles (8.3395, 9.1553) (8.4846, 9.1941) (8.5688, 9.2552) (8.6121, 9.3531) knots 0 0 0 0 1 1 1 1
  spline S437 degree 3 poles (5.1346, 0.839) (4.6392, 0.9696) (4.1389, 1.3506) (4.1389, 1.5972) knots 0 0 0 0 1 1 1 1
  spline S438 degree 3 poles (10.0627, 6.2334) (9.9429, 6.5182) (9.7174, 6.8169) (9.5037, 6.9737) knots 0 0 0 0 1 1 1 1
  spline S439 degree 3 poles (9.5037, 6.9737) (9.3593, 7.0797) (9.3292, 7.1436) (9.3119, 7.3814) knots 0 0 0 0 1 1 1 1
  spline S440 degree 3 poles (5.8327, 11.1553) (5.8977, 11.3318) (6.0662, 11.6123) (6.2046, 11.7743) knots 0 0 0 0 1 1 1 1
  spline S441 degree 3 poles (5.578, 2.1276) (6.2235, 2.1274) (6.8007, 1.9328) (6.8522, 1.698) knots 0 0 0 0 1 1 1 1
  spline S442 degree 3 poles (9.3119, 7.3814) (9.2835, 7.771) (9.2105, 8.0439) (9.0615, 8.3174) knots 0 0 0 0 1 1 1 1
  spline S443 degree 3 poles (6.1124, 12.0526) (5.9025, 11.8948) (5.6467, 11.5072) (5.5602, 11.2158) knots 0 0 0 0 1 1 1 1
  spline S444 degree 3 poles (7.8879, 11.1002) (8.2257, 11.2952) (8.2251, 11.297) (7.8714, 11.1457) knots 0 0 0 0 1 1 1 1
  spline S445 degree 3 poles (4.4338, 1.9054) (4.7393, 2.0533) (5.1225, 2.1277) (5.578, 2.1276) knots 0 0 0 0 1 1 1 1
  spline S446 degree 3 poles (8.738, 12.3312) (8.6701, 12.3905) (8.6131, 12.4096) (8.5039, 12.4097) knots 0 0 0 0 1 1 1 1
  spline S447 degree 3 poles (9.6995, 11.0543) (9.6895, 11.1388) (9.6959, 11.1692) (9.7397, 11.2439) knots 0 0 0 0 1 1 1 1
  spline S448 degree 3 poles (9.0186, 9.7228) (9.0374, 9.7773) (9.0815, 9.831) (9.1579, 9.8924) knots 0 0 0 0 1 1 1 1
  spline S449 degree 3 poles (6.4852, 12.226) (6.4182, 12.1574) (6.3938, 12.1454) (6.3212, 12.1454) knots 0 0 0 0 1 1 1 1
  spline S450 degree 3 poles (4.1379, 1.0234) (4.402, 0.7792) (4.7633, 0.5846) (5.0838, 0.5141) knots 0 0 0 0 1 1 1 1
  spline S451 degree 3 poles (9.4479, 12.1081) (9.3707, 12.1095) (9.3367, 12.1223) (9.2813, 12.1708) knots 0 0 0 0 1 1 1 1
  spline S452 degree 3 poles (7.8714, 11.1457) (7.3441, 10.9202) (6.8433, 10.6359) (6.4382, 10.332) knots 0 0 0 0 1 1 1 1
  spline S453 degree 3 poles (10.2085, 5.6081) (10.1951, 5.8439) (10.1559, 6.0119) (10.0627, 6.2334) knots 0 0 0 0 1 1 1 1
  spline S454 degree 3 poles (6.4902, 10.1039) (6.7798, 10.3908) (7.2938, 10.7572) (7.8879, 11.1002) knots 0 0 0 0 1 1 1 1
  spline S455 degree 3 poles (6.2046, 11.7743) (6.2878, 11.8717) (6.3538, 11.9106) (6.3538, 11.8623) knots 0 0 0 0 1 1 1 1
  spline S456 degree 3 poles (8.296, 12.4605) (8.1795, 12.5195) (8.1272, 12.5227) (7.9821, 12.4796) knots 0 0 0 0 1 1 1 1
  spline S457 degree 3 poles (9.7397, 11.2439) (9.8029, 11.3518) (9.8058, 11.4412) (9.7496, 11.5514) knots 0 0 0 0 1 1 1 1
  spline S458 degree 3 poles (4.8843, 12.0613) (4.7955, 12.1297) (4.759, 12.1454) (4.6885, 12.1454) knots 0 0 0 0 1 1 1 1
  line L49 (3.8239, 9.279) -> (3.8239, 9.279)
  spline S459 degree 3 poles (6.5695, 11.9187) (6.6651, 12.021) (6.7562, 12.1048) (6.772, 12.1048) knots 0 0 0 0 1 1 1 1
  spline S460 degree 3 poles (6.772, 12.1048) (6.7909, 12.1048) (6.8009, 12.082) (6.8011, 12.0387) knots 0 0 0 0 1 1 1 1
  spline S461 degree 3 poles (7.8084, 12.4898) (7.7205, 12.5441) (7.6436, 12.5424) (7.4851, 12.4828) knots 0 0 0 0 1 1 1 1
  spline S462 degree 3 poles (6.8011, 12.0387) (6.8013, 12.0024) (6.8106, 11.959) (6.8218, 11.9422) knots 0 0 0 0 1 1 1 1
  spline S463 degree 3 poles (6.8218, 11.9422) (6.839, 11.9165) (6.8487, 11.9204) (6.8834, 11.9666) knots 0 0 0 0 1 1 1 1
  spline S464 degree 3 poles (9.2813, 12.1708) (9.1805, 12.259) (9.0886, 12.2908) (8.9223, 12.2949) knots 0 0 0 0 1 1 1 1
  spline S465 degree 3 poles (6.8834, 11.9666) (6.9274, 12.0252) (7.1583, 12.2064) (7.1889, 12.2064) knots 0 0 0 0 1 1 1 1
  spline S466 degree 3 poles (8.2435, 9.1046) (8.2435, 9.1184) (8.2867, 9.1412) (8.3395, 9.1553) knots 0 0 0 0 1 1 1 1
  spline S467 degree 3 poles (9.4502, 10.359) (9.5401, 10.4589) (9.5787, 10.5644) (9.554, 10.6423) knots 0 0 0 0 1 1 1 1
  spline S468 degree 3 poles (9.1579, 9.8924) (9.2726, 9.9845) (9.3611, 10.1234) (9.3611, 10.2113) knots 0 0 0 0 1 1 1 1
  spline S469 degree 3 poles (9.8442, 4.434) (10.1184, 4.8041) (10.2332, 5.174) (10.2085, 5.6081) knots 0 0 0 0 1 1 1 1
  spline S470 degree 3 poles (2.9908, 1.6908) (3.3054, 1.467) (3.6474, 1.2767) (3.9052, 1.182) knots 0 0 0 0 1 1 1 1
  spline S471 degree 3 poles (9.3611, 10.2113) (9.3611, 10.24) (9.3974, 10.3002) (9.4502, 10.359) knots 0 0 0 0 1 1 1 1
  spline S472 degree 3 poles (9.7388, 11.7223) (9.8154, 11.936) (9.6891, 12.1035) (9.4479, 12.1081) knots 0 0 0 0 1 1 1 1
  spline S473 degree 3 poles (8.4213, 8.9643) (8.3235, 9.0277) (8.2435, 9.0909) (8.2435, 9.1046) knots 0 0 0 0 1 1 1 1
  spline S474 degree 3 poles (7.2193, 12.0182) (7.2259, 12.0115) (7.2877, 12.0476) (7.3564, 12.0982) knots 0 0 0 0 1 1 1 1
  spline S475 degree 3 poles (9.3002, 10.5655) (9.3002, 10.525) (9.1768, 10.4083) (8.9991, 10.2805) knots 0 0 0 0 1 1 1 1
  spline S476 degree 3 poles (8.2775, 9.5445) (8.2683, 9.5361) (8.2889, 9.5194) (8.3233, 9.5074) knots 0 0 0 0 1 1 1 1
  spline S477 degree 3 poles (1.5005, 3.286) (1.4774, 3.3921) (1.4257, 3.57) (1.3854, 3.6813) knots 0 0 0 0 1 1 1 1
  spline S478 degree 3 poles (9.2583, 11.8609) (9.407, 11.8609) (9.5061, 11.8526) (9.5142, 11.8394) knots 0 0 0 0 1 1 1 1
  line L50 (6.3959, 11.7325) -> (6.5695, 11.9187)
  spline S479 degree 3 poles (9.3264, 11.0128) (9.3912, 11.0174) (9.449, 11.0133) (9.4548, 11.0038) knots 0 0 0 0 1 1 1 1
  line L51 (6.3748, 11.7879) -> (6.3959, 11.7325)
  spline S480 degree 3 poles (5.2057, 0.4341) (4.8057, 0.4977) (4.4091, 0.6918) (4.1103, 0.9702) knots 0 0 0 0 1 1 1 1
  spline S481 degree 3 poles (7.1522, 12.1052) (7.1606, 12.137) (7.1408, 12.1277) (7.0639, 12.0632) knots 0 0 0 0 1 1 1 1
  spline S482 degree 3 poles (8.0245, 9.354) (7.8017, 9.3293) (7.7494, 9.3009) (7.8457, 9.257) knots 0 0 0 0 1 1 1 1
  spline S483 degree 3 poles (7.2421, 11.9625) (7.1966, 11.9625) (7.1389, 12.0541) (7.1522, 12.1052) knots 0 0 0 0 1 1 1 1
  spline S484 degree 3 poles (7.328, 12.0112) (7.2995, 11.9844) (7.2608, 11.9625) (7.2421, 11.9625) knots 0 0 0 0 1 1 1 1
  spline S485 degree 3 poles (7.3564, 12.0982) (7.6214, 12.2933) (7.7703, 12.3271) (7.6503, 12.1648) knots 0 0 0 0 1 1 1 1
  spline S486 degree 3 poles (8.9989, 10.2112) (9.1301, 10.2017) (9.1247, 10.1541) (8.9813, 10.0568) knots 0 0 0 0 1 1 1 1
  spline S487 degree 3 poles (6.9146, 11.9206) (6.887, 11.8878) (6.8561, 11.8609) (6.8459, 11.8609) knots 0 0 0 0 1 1 1 1
  spline S488 degree 3 poles (9.2433, 10.5948) (9.2904, 10.6042) (9.3002, 10.5992) (9.3002, 10.5655) knots 0 0 0 0 1 1 1 1
  spline S489 degree 3 poles (6.8459, 11.8609) (6.8116, 11.8609) (6.7636, 11.9316) (6.7568, 11.9922) knots 0 0 0 0 1 1 1 1
  spline S490 degree 3 poles (6.7568, 11.9922) (6.7502, 12.0508) (6.7458, 12.0476) (6.5887, 11.8703) knots 0 0 0 0 1 1 1 1
  spline S491 degree 3 poles (0.7839, 5.0741) (0.7204, 5.3143) (0.7197, 5.6809) (0.7822, 5.9337) knots 0 0 0 0 1 1 1 1
  spline S492 degree 3 poles (6.3996, 11.6814) (6.3838, 11.6776) (6.3616, 11.7017) (6.3481, 11.7375) knots 0 0 0 0 1 1 1 1
  spline S493 degree 3 poles (6.5887, 11.8703) (6.5, 11.7701) (6.4149, 11.6852) (6.3996, 11.6814) knots 0 0 0 0 1 1 1 1
  spline S494 degree 3 poles (8.5178, 12.0604) (8.4544, 11.9851) (8.4526, 11.9536) (8.5128, 11.9711) knots 0 0 0 0 1 1 1 1
  spline S495 degree 3 poles (6.3481, 11.7375) (6.3351, 11.7721) (6.315, 11.7973) (6.3035, 11.7935) knots 0 0 0 0 1 1 1 1
  line L52 (8.0525, 12.1442) -> (8.1054, 12.207)
  spline S496 degree 3 poles (1.2638, 4.0692) (1.2237, 4.2238) (1.1962, 4.2818) (1.0995, 4.4155) knots 0 0 0 0 1 1 1 1
  spline S497 degree 3 poles (9.4548, 11.0038) (9.4725, 10.9753) (9.3917, 10.8629) (9.261, 10.7342) knots 0 0 0 0 1 1 1 1
  spline S498 degree 3 poles (7.757, 12.1239) (7.8873, 12.1951) (8.1044, 12.258) (8.1541, 12.2389) knots 0 0 0 0 1 1 1 1
  spline S499 degree 3 poles (9.5439, 11.3885) (9.5436, 11.3418) (9.466, 11.2423) (9.3368, 11.1228) knots 0 0 0 0 1 1 1 1
  spline S500 degree 3 poles (1.3854, 3.6813) (1.345, 3.7926) (1.2904, 3.9671) (1.2638, 4.0692) knots 0 0 0 0 1 1 1 1
  spline S501 degree 3 poles (7.0639, 12.0632) (7.0094, 12.0176) (6.9422, 11.9534) (6.9146, 11.9206) knots 0 0 0 0 1 1 1 1
  spline S502 degree 3 poles (3.763, 1.1797) (3.5156, 1.2838) (3.1909, 1.47) (2.9348, 1.6546) knots 0 0 0 0 1 1 1 1
  spline S503 degree 3 poles (9.0157, 11.8781) (9.0157, 11.8687) (9.1249, 11.8609) (9.2583, 11.8609) knots 0 0 0 0 1 1 1 1
  spline S504 degree 3 poles (9.0335, 12.0311) (9.1067, 12.0165) (9.1141, 11.9844) (9.0563, 11.9321) knots 0 0 0 0 1 1 1 1
  spline S505 degree 3 poles (9.4776, 11.7425) (9.4183, 11.6529) (9.3516, 11.5234) (9.3319, 11.4596) knots 0 0 0 0 1 1 1 1
  spline S506 degree 3 poles (8.5128, 11.9711) (8.7316, 12.0349) (8.9112, 12.0556) (9.0335, 12.0311) knots 0 0 0 0 1 1 1 1
  spline S507 degree 3 poles (9.261, 10.7342) (9.1345, 10.6094) (9.1297, 10.5721) (9.2433, 10.5948) knots 0 0 0 0 1 1 1 1
  spline S508 degree 3 poles (4.1103, 0.9702) (4.0113, 1.0625) (3.9418, 1.1044) (3.763, 1.1797) knots 0 0 0 0 1 1 1 1
  spline S509 degree 3 poles (9.0563, 11.9321) (9.034, 11.9118) (9.0157, 11.8876) (9.0157, 11.8781) knots 0 0 0 0 1 1 1 1
  spline S510 degree 3 poles (9.4309, 11.4139) (9.5079, 11.4139) (9.544, 11.4058) (9.5439, 11.3885) knots 0 0 0 0 1 1 1 1
  line L53 (8.9991, 10.2805) -> (8.9114, 10.2175)
  line L54 (8.9114, 10.2175) -> (8.9989, 10.2112)
  spline S511 degree 3 poles (8.1541, 12.2389) (8.1848, 12.2271) (8.181, 12.2169) (8.125, 12.159) knots 0 0 0 0 1 1 1 1
  spline S512 degree 3 poles (9.5142, 11.8394) (9.5216, 11.8276) (9.505, 11.784) (9.4776, 11.7425) knots 0 0 0 0 1 1 1 1
  spline S513 degree 3 poles (7.1889, 12.2064) (7.199, 12.2064) (7.2072, 12.1668) (7.2072, 12.1183) knots 0 0 0 0 1 1 1 1
  line L55 (9.2087, 11.0044) -> (9.3264, 11.0128)
  spline S514 degree 3 poles (8.776, 9.7781) (8.7792, 9.7465) (8.6356, 9.6724) (8.4569, 9.6134) knots 0 0 0 0 1 1 1 1
  spline S515 degree 3 poles (6.437, 9.7543) (6.3375, 9.9623) (6.3357, 9.9508) (6.4902, 10.1039) knots 0 0 0 0 1 1 1 1
  spline S516 degree 3 poles (2.9348, 1.6546) (2.8426, 1.7209) (2.7062, 1.8034) (2.6316, 1.8379) knots 0 0 0 0 1 1 1 1
  spline S517 degree 3 poles (8.3233, 9.5074) (8.4769, 9.4539) (8.3533, 9.3904) (8.0245, 9.354) knots 0 0 0 0 1 1 1 1
  spline S518 degree 3 poles (2.6316, 1.8379) (2.0666, 2.099) (1.6392, 2.6462) (1.5005, 3.286) knots 0 0 0 0 1 1 1 1
  spline S519 degree 3 poles (8.125, 12.159) (8.0538, 12.0856) (8.039, 12.0311) (8.0962, 12.0532) knots 0 0 0 0 1 1 1 1
  spline S520 degree 3 poles (7.6503, 12.1648) (7.5801, 12.0698) (7.626, 12.0522) (7.757, 12.1239) knots 0 0 0 0 1 1 1 1
  spline S521 degree 3 poles (8.6866, 9.8203) (8.7347, 9.8083) (8.7749, 9.7893) (8.776, 9.7781) knots 0 0 0 0 1 1 1 1
  spline S522 degree 3 poles (8.4569, 9.6134) (8.3675, 9.5839) (8.2868, 9.5529) (8.2775, 9.5445) knots 0 0 0 0 1 1 1 1
  spline S523 degree 3 poles (8.4924, 12.1548) (8.5839, 12.1701) (8.5903, 12.1465) (8.5178, 12.0604) knots 0 0 0 0 1 1 1 1
  spline S524 degree 3 poles (7.2072, 12.1183) (7.2072, 12.0699) (7.2126, 12.0248) (7.2193, 12.0182) knots 0 0 0 0 1 1 1 1
  spline S525 degree 3 poles (8.0962, 12.0532) (8.1531, 12.0751) (8.4092, 12.1408) (8.4924, 12.1548) knots 0 0 0 0 1 1 1 1
  line L56 (9.3368, 11.1228) -> (9.2087, 11.0044)
  spline S526 degree 3 poles (8.9813, 10.0568) (8.9164, 10.0128) (8.8038, 9.9465) (8.7312, 9.9095) knots 0 0 0 0 1 1 1 1
  spline S527 degree 3 poles (9.3319, 11.4596) (9.3184, 11.416) (9.3229, 11.4139) (9.4309, 11.4139) knots 0 0 0 0 1 1 1 1
  spline S528 degree 3 poles (1.0995, 4.4155) (0.9555, 4.6146) (0.8436, 4.8481) (0.7839, 5.0741) knots 0 0 0 0 1 1 1 1
  spline S529 degree 3 poles (7.4991, 9.1799) (6.9868, 9.2296) (6.5837, 9.4476) (6.437, 9.7543) knots 0 0 0 0 1 1 1 1
  spline S530 degree 3 poles (0.7822, 5.9337) (0.8927, 6.3804) (1.1472, 6.7875) (1.4592, 7.0165) knots 0 0 0 0 1 1 1 1
  spline S531 degree 3 poles (8.0505, 11.1301) (7.3735, 10.756) (6.8792, 10.4129) (6.5316, 10.0756) knots 0 0 0 0 1 1 1 1
  spline S532 degree 3 poles (6.4147, 9.9356) (6.4147, 9.9011) (6.5085, 9.716) (6.5645, 9.64) knots 0 0 0 0 1 1 1 1
  spline S533 degree 3 poles (6.3035, 11.7935) (6.2526, 11.7769) (6.0609, 11.508) (5.9678, 11.3225) knots 0 0 0 0 1 1 1 1
  line L57 (8.1054, 12.207) -> (7.956, 12.1534)
  spline S534 degree 3 poles (8.5107, 11.419) (8.5339, 11.3958) (8.5527, 11.4076) (8.0505, 11.1301) knots 0 0 0 0 1 1 1 1
  spline S535 degree 3 poles (6.3867, 10.3581) (6.803, 10.6716) (7.3362, 10.9727) (7.8879, 11.2061) knots 0 0 0 0 1 1 1 1
  line L58 (6.1089, 10.2462) -> (6.1789, 10.2018)
  spline S536 degree 3 poles (5.837, 10.5825) (5.8713, 10.4667) (5.9874, 10.3232) (6.1089, 10.2462) knots 0 0 0 0 1 1 1 1
  spline S537 degree 3 poles (7.8879, 11.2061) (8.3088, 11.3841) (8.4853, 11.4444) (8.5107, 11.419) knots 0 0 0 0 1 1 1 1
  spline S538 degree 3 poles (7.6421, 9.2212) (7.7965, 9.2194) (7.8015, 9.2208) (7.7691, 9.2565) knots 0 0 0 0 1 1 1 1
  spline S539 degree 3 poles (5.9678, 11.3225) (5.8079, 11.0039) (5.7721, 10.8011) (5.837, 10.5825) knots 0 0 0 0 1 1 1 1
  spline S540 degree 3 poles (6.5316, 10.0756) (6.4673, 10.0133) (6.4147, 9.9503) (6.4147, 9.9356) knots 0 0 0 0 1 1 1 1
  line L59 (6.1789, 10.2018) -> (6.3867, 10.3581)
  spline S541 degree 3 poles (6.5645, 9.64) (6.7352, 9.4081) (7.2034, 9.2261) (7.6421, 9.2212) knots 0 0 0 0 1 1 1 1
extrude "Extrude24" cut sketch "rpi3" against normal blind 0.05 bodies 14
named bodies: "Board", "CPU", "HDMI", "USB", "Memory"
